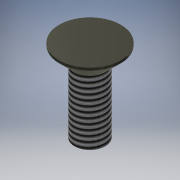
# Autodesk Inventor part: SB　8mm皿ネジ
Saved by Autodesk Inventor 2020.2 (Build 242310000, 310)
## iProperties
Created: 2014-02-15
Part Number: SB　8mm皿ネジ
Material: Steel, Mild
Document SubType Name: Modeling
Designer: shiota
Mass: 0.59726 g
Surface Area: 1.2895 cm^2
Volume: 0.0759873 cm^3
Density: 7.86 g/cm^3
Appearance: ガンメタル
Author: shiota
Autodesk Inventor part; units mm, degrees
ref_plane "YZ Plane" through (0, 0, 0) normal (1, 0, 0) x (0, 1, 0)
ref_plane "XZ Plane" through (0, 0, 0) normal (0, 1, 0) x (-1, 0, 0)
ref_plane "XY Plane" through (0, 0, 0) normal (0, 0, 1) x (1, 0, 0)
sketch "スケッチ1" plane through (0, 0, 0) normal (0, 0, 1) x (1, 0, 0)
  circle A0 centre (0, 0) radius 1.5
  dimension "d0" = 3
  constraints: 1 centre point, 1 coincident
  measures "d0" diameter of A0
extrude "押し出し1" add sketch "スケッチ1" along normal blind 6.25
sketch "スケッチ2" plane through (0, 0, 6.25) normal (0, 0, 1) x (1, 0, 0)
  circle A0 centre (0, 0) radius 1.5 projected
  circle A1 centre (0, 0) radius 3
  dimension "d3" = 6
  constraints: 1 centre point, 1 coincident
  measures "d3" diameter of A1
extrude "押し出し2" add sketch "スケッチ2" along normal blind 1.75 contours A0 | A1
thread "ねじ1" size "M3x0.5" class "6g" standard "ANSI Metric M Profile" full length
chamfer "面取り1" distance 1.5 angle 45 1 edges at (-3, 0, 6.25)
